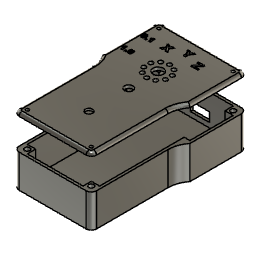
3018 pendant case (Autodesk Fusion 360 design; units mm, degrees)
Autodesk Fusion 360 part; units mm, degrees
note: some values were not read from the file. Chosen so that the rebuilt part matches the saved one: the layout of a text. Set by a fixed rule: which sketch regions a step uses.
sketch "Sketch1" plane through (0, 0, 0) normal (0, 0, 1) x (1, 0, 0)
  line L0 (35, -45) -> (-35, -45)
  line L1 (-35, -45) -> (-35, 45)
  line L2 (35, 45) -> (35, -45)
  line L3 (35, -45) -> (-35, 45) construction
  line L4 (-35, -45) -> (35, 45) construction
  line L5 (-35, 45) -> (-39.456, 45)
  line L6 (-39.456, 45) -> (-39.456, 95)
  line L7 (-39.456, 95) -> (40.544, 95)
  line L8 (40.544, 95) -> (40.544, 45)
  line L9 (40.544, 45) -> (35, 45)
  line L10 (43.044, 42.5) -> (37.5, 42.5)
  line L11 (37.5, 42.5) -> (37.5, -47.5)
  line L12 (37.5, -47.5) -> (-37.5, -47.5)
  line L13 (-37.5, -47.5) -> (-37.5, 42.5)
  line L14 (-37.5, 42.5) -> (-41.956, 42.5)
  line L15 (-41.956, 42.5) -> (-41.956, 97.5)
  line L16 (-41.956, 97.5) -> (43.044, 97.5)
  line L17 (43.044, 97.5) -> (43.044, 42.5)
  dimension "d2" = 90
  dimension "d4" = 50
  dimension "d5" = 80
  dimension "d6" = 50
  dimension "d7" = -2.5
  dimension "d160" = 70
  constraint horizontal L0
  constraint perpendicular L0 L1
  constraint parallel L1 L2
  constraint coincident L3 origin
  constraint coincident L4 origin
  constraint perpendicular L1 L5
  constraint perpendicular L6 L7
  constraint perpendicular L7 L8
  constraint perpendicular L2 L9
  constraint perpendicular L8 L9
  measures "d2" distance of L0.end L1.end
  measures "d4" distance of L5.end L6.end
  measures "d5" distance of L6.end L7.end
  measures "d6" distance of L7.end L8.end
  measures "d160" distance of L0.start L0.end
extrude "Extrude1" add sketch "Sketch1" along normal blind 2 contours L0 L1 L2 L5 L6 L7 L8 L9 makes body 1
extrude "Extrude2" add sketch "Sketch1" along normal blind 32 bodies 1
sketch "Sketch2" plane through (0, 0, 2) normal (0, 0, 1) x (-1, 0, 0)
  line L0 (-40.544, -45) -> (-40.544, -95)
  line L1 (-40.544, -95) -> (39.456, -95)
  line L2 (39.456, -95) -> (39.456, -45)
  line L3 (39.456, -45) -> (35, -45)
  line L4 (35, -45) -> (35, 45)
  line L5 (35, 45) -> (-35, 45)
  line L6 (-35, 45) -> (-35, -45)
  line L7 (-35, -45) -> (-40.544, -45)
  circle A0 centre (0, 10) radius 32.5
  line L8 (39.456, -95) -> (31.456, -95)
  line L9 (31.456, -95) -> (31.456, -87)
  line L10 (31.456, -87) -> (39.456, -87)
  line L11 (39.456, -87) -> (39.456, -95)
  line L12 (-40.544, -95) -> (-32.544, -95)
  line L13 (-32.544, -95) -> (-32.544, -87)
  line L14 (-32.544, -87) -> (-40.544, -87)
  line L15 (-40.544, -87) -> (-40.544, -95)
  line L16 (35, 45) -> (27, 45)
  line L17 (27, 45) -> (27, 37)
  line L18 (27, 37) -> (35, 37)
  line L19 (35, 37) -> (35, 45)
  line L20 (-35, 45) -> (-27, 45)
  line L21 (-27, 45) -> (-27, 37)
  line L22 (-27, 37) -> (-35, 37)
  line L23 (-35, 37) -> (-35, 45)
  dimension "d13" = 65
  dimension "d24" = 8
  dimension "d25" = 8
  dimension "d26" = 8
  dimension "d27" = 8
  dimension "d28" = 8
  dimension "d29" = 8
  dimension "d30" = 8
  dimension "d31" = 8
  constraint horizontal L8
  constraint vertical L9
  constraint horizontal L10
  constraint vertical L11
  constraint coincident L1.end L2.start
  constraint horizontal L12
  constraint vertical L13
  constraint horizontal L14
  constraint vertical L15
  constraint coincident L0.end L1.start
  constraint horizontal L16
  constraint vertical L17
  constraint horizontal L18
  constraint vertical L19
  constraint coincident L4.end L5.start
  constraint horizontal L20
  constraint vertical L21
  constraint horizontal L22
  constraint vertical L23
  constraint coincident L5.end L6.start
  measures "d13" diameter of A0
  measures "d24" distance of L1.end L8.end
  measures "d25" distance of L1.end L10.end
  measures "d26" distance of L0.end L12.end
  measures "d27" distance of L0.end L14.end
  measures "d28" distance of L4.end L16.end
  measures "d29" distance of L4.end L18.end
  measures "d30" distance of L5.end L20.end
  measures "d31" distance of L5.end L22.end
extrude "Extrude3" add sketch "Sketch2" along normal up to surface (30 mm away) contours L0 L1 L12 L13 L14 L15 | L5 L6 L20 L21 L22 L23 | L1 L2 L8 L9 L10 L11 | L4 L5 L16 L17 L18 L19 bodies 1
fillet "Fillet1" radius 5 4 edges at (37.5, -47.5, 16) (-37.5, -47.5, 16) (43.044, 97.5, 16) (-41.956, 97.5, 16) on bodies 1
fillet "Fillet7" radius 25 2 edges at (-37.5, 42.5, 16) (37.5, 42.5, 16) on bodies 1
fillet "Fillet2" [suppressed]
fillet "Fillet3" [suppressed]
sketch "Sketch3" plane through (0, 0, 32) normal (0, 0, 1) x (-1, 0, 0)
  arc A0 (36.956, -97.5) -> (41.956, -92.5) centre (36.956, -92.5) ccw
  line L0 (41.956, -92.5) -> (41.956, -42.5)
  line L1 (37.5, -42.5) -> (37.5, 42.5)
  arc A1 (37.5, 42.5) -> (32.5, 47.5) centre (32.5, 42.5) ccw
  line L2 (32.5, 47.5) -> (-32.5, 47.5)
  arc A2 (-32.5, 47.5) -> (-37.5, 42.5) centre (-32.5, 42.5) ccw
  line L3 (-37.5, 42.5) -> (-37.5, -42.5)
  line L4 (-43.044, -42.5) -> (-43.044, -92.5)
  arc A3 (-43.044, -92.5) -> (-38.044, -97.5) centre (-38.044, -92.5) ccw
  line L5 (-38.044, -97.5) -> (36.956, -97.5)
  line L6 (-40.544, -87) -> (-40.544, -45)
  line L7 (-40.544, -45) -> (-35, -45)
  line L8 (-35, -45) -> (-35, 37)
  line L9 (-35, 37) -> (-27, 37)
  line L10 (-27, 37) -> (-27, 45)
  line L11 (-27, 45) -> (27, 45)
  line L12 (27, 45) -> (27, 37)
  line L13 (27, 37) -> (35, 37)
  line L14 (35, 37) -> (35, -45)
  line L15 (35, -45) -> (39.456, -45)
  line L16 (39.456, -45) -> (39.456, -87)
  line L17 (39.456, -87) -> (31.456, -87)
  line L18 (31.456, -87) -> (31.456, -95)
  line L19 (31.456, -95) -> (-32.544, -95)
  line L20 (-32.544, -95) -> (-32.544, -87)
  line L21 (-32.544, -87) -> (-40.544, -87)
  circle A4 centre (35.456, -91) radius 2.5
  circle A5 centre (-36.544, -91) radius 2.5
  circle A6 centre (31, 41) radius 2.5
  circle A7 centre (-31, 41) radius 2.5
  line L22 (41.956, -42.5) -> (37.5, -42.5)
  line L23 (-37.5, -42.5) -> (-43.044, -42.5)
  dimension "d34" = 5
  dimension "d35" = 4
  dimension "d36" = 4
  dimension "d37" = 5
  dimension "d38" = 4
  dimension "d39" = 4
  dimension "d40" = 5
  dimension "d41" = 4
  dimension "d42" = 4
  dimension "d43" = 5
  dimension "d44" = 4
  dimension "d45" = 4
  measures "d34" diameter of A4
  measures "d35" distance of L17 A4.centre
  measures "d36" distance of L18 A4.centre
  measures "d37" diameter of A5
  measures "d38" distance of L20 A5.centre
  measures "d39" distance of L21 A5.centre
  measures "d40" diameter of A6
  measures "d41" distance of L13 A6.centre
  measures "d42" distance of L12 A6.centre
  measures "d43" diameter of A7
  measures "d44" distance of L10 A7.centre
  measures "d45" distance of L9 A7.centre
extrude "Extrude4" cut sketch "Sketch3" against normal blind 5.2 contours A4 | A5 | A6 | A7 bodies 1
ref_plane "WorkPlane1" through (0.544, 25, 62) normal (0, 0, 1) x (1, 0, 0)
sketch "Sketch4" plane through (0, 25, 62) normal (0, 0, 1) x (1, 0, 0)
  arc A0 (-36.956, 72.5) -> (-41.956, 67.5) centre (-36.956, 67.5) ccw
  line L0 (-36.956, 72.5) -> (38.044, 72.5)
  arc A1 (43.044, 67.5) -> (38.044, 72.5) centre (38.044, 67.5) ccw
  line L1 (43.044, 67.5) -> (43.044, 17.5)
  line L2 (37.5, 1.8009) -> (37.5, -67.5)
  arc A2 (32.5, -72.5) -> (37.5, -67.5) centre (32.5, -67.5) ccw
  line L3 (32.5, -72.5) -> (-32.5, -72.5)
  arc A3 (-37.5, -67.5) -> (-32.5, -72.5) centre (-32.5, -67.5) ccw
  line L4 (-37.5, -67.5) -> (-37.5, 3.2541)
  line L5 (-41.956, 17.5) -> (-41.956, 67.5)
  arc A4 (43.044, 17.5) -> (37.5, 1.8009) centre (62.5, 1.8009) ccw
  arc A5 (-37.5, 3.2541) -> (-41.956, 17.5) centre (-62.5, 3.2541) ccw
extrude "Extrude5" add sketch "Sketch4" along normal blind 3 separate body makes body 2
sketch "Sketch5" plane through (0, 0, 32) normal (0, 0, 1) x (1, 0, 0)
  circle A0 centre (36.544, 91) radius 2.5
  circle A1 centre (-35.456, 91) radius 2.5
  circle A2 centre (31, -41) radius 2.5
  circle A3 centre (-31, -41) radius 2.5
  circle A4 centre (-35.456, 91) radius 1.5
  circle A5 centre (36.544, 91) radius 1.5
  circle A6 centre (31, -41) radius 1.5
  circle A7 centre (-31, -41) radius 1.5
  circle A8 centre (36.544, 91) radius 2.5
  circle A9 centre (-31, -41) radius 2.5
  circle A10 centre (-35.456, 91) radius 2.5
  circle A11 centre (31, -41) radius 2.5
  arc A12 (-36.956, 97.5) -> (-41.956, 92.5) centre (-36.956, 92.5) ccw
  line L0 (-41.956, 92.5) -> (-41.956, 42.5)
  arc A13 (-37.5, 28.2541) -> (-41.956, 42.5) centre (-62.5, 28.2541) ccw
  line L1 (-37.5, 28.2541) -> (-37.5, -42.5)
  arc A14 (-37.5, -42.5) -> (-32.5, -47.5) centre (-32.5, -42.5) ccw
  line L2 (-32.5, -47.5) -> (32.5, -47.5)
  arc A15 (32.5, -47.5) -> (37.5, -42.5) centre (32.5, -42.5) ccw
  line L3 (37.5, -42.5) -> (37.5, 26.8009)
  arc A16 (43.044, 42.5) -> (37.5, 26.8009) centre (62.5, 26.8009) ccw
  line L4 (43.044, 42.5) -> (43.044, 92.5)
  arc A17 (43.044, 92.5) -> (38.044, 97.5) centre (38.044, 92.5) ccw
  line L5 (38.044, 97.5) -> (-36.956, 97.5)
  line L6 (40.544, 87) -> (40.544, 45)
  line L7 (40.544, 45) -> (35, 45)
  line L8 (35, 45) -> (35, -37)
  line L9 (35, -37) -> (27, -37)
  line L10 (27, -37) -> (27, -45)
  line L11 (27, -45) -> (-27, -45)
  line L12 (-27, -45) -> (-27, -37)
  line L13 (-27, -37) -> (-35, -37)
  line L14 (-35, -37) -> (-35, 45)
  line L15 (-35, 45) -> (-39.456, 45)
  line L16 (-39.456, 45) -> (-39.456, 87)
  line L17 (-39.456, 87) -> (-31.456, 87)
  line L18 (-31.456, 87) -> (-31.456, 95)
  line L19 (-31.456, 95) -> (32.544, 95)
  line L20 (32.544, 95) -> (32.544, 87)
  line L21 (32.544, 87) -> (40.544, 87)
  dimension "d141" = 3
  dimension "d142" = 3
  dimension "d143" = 3
  dimension "d144" = 3
  constraint concentric A1 A4
  constraint concentric A0 A5
  constraint concentric A2 A6
  constraint concentric A3 A7
  measures "d141" diameter of A4
  measures "d142" diameter of A5
  measures "d143" diameter of A6
  measures "d144" diameter of A7
extrude "Extrude7" cut sketch "Sketch5" along normal up to surface (33 mm away) contours A4 | A5 | A6 | A7 bodies 2
sketch "Sketch6" plane through (0, 0, 65) normal (0, 0, 1) x (-1, 0, 0)
  circle A0 centre (0, 12.2844) radius 30.6
  circle A1 centre (0, 12.2844) radius 33.6
  circle A2 centre (0, 12.2844) radius 3.5
  circle A3 centre (-31, 41) radius 1.5
  circle A4 centre (-36.544, -91) radius 1.5
  circle A5 centre (31, 41) radius 1.5
  circle A6 centre (35.456, -91) radius 1.5
  arc A7 (37.5, 42.5) -> (32.5, 47.5) centre (32.5, 42.5) ccw
  line L0 (32.5, 47.5) -> (-32.5, 47.5)
  arc A8 (-32.5, 47.5) -> (-37.5, 42.5) centre (-32.5, 42.5) ccw
  line L1 (-37.5, 42.5) -> (-37.5, -26.8009)
  arc A9 (-43.044, -42.5) -> (-37.5, -26.8009) centre (-62.5, -26.8009) ccw
  line L2 (-43.044, -42.5) -> (-43.044, -92.5)
  arc A10 (-43.044, -92.5) -> (-38.044, -97.5) centre (-38.044, -92.5) ccw
  line L3 (-38.044, -97.5) -> (36.956, -97.5)
  arc A11 (36.956, -97.5) -> (41.956, -92.5) centre (36.956, -92.5) ccw
  line L4 (41.956, -92.5) -> (41.956, -42.5)
  arc A12 (37.5, -28.2541) -> (41.956, -42.5) centre (62.5, -28.2541) ccw
  line L5 (37.5, -28.2541) -> (37.5, 42.5)
  dimension "d57" = 61.2
  dimension "d58" = 3
  dimension "d62" = 7
  constraint concentric A0 A2
  measures "d57" diameter of A0
  measures "d62" diameter of A2
fillet "Fillet6" radius 3 12 edges at (-38.64, 35.7174, 65) (-37.5, -7.123, 65) (-36.0355, -46.0355, 65) (0, -47.5, 65) (36.0355, -46.0355, 65) (37.5, -7.8496, 65) (38.9267, 35.1255, 65) (43.044, 67.5, 65) (41.5795, 96.0355, 65) (0.544, 97.5, 65) (-40.4916, 96.0355, 65) (-41.956, 67.5, 65) on bodies 2
sketch "Sketch10" plane through (0, 0, 0) normal (0, 0, -1) x (1, 0, 0)
  line L0 (-47.5, -83.9701, -14.6252) -> (-47.5, -71.3701, -14.6252)
  line L1 (-47.5, -71.3701, -14.6252) -> (-47.5, -71.3701, -27.2252)
  line L2 (-47.5, -71.3701, -27.2252) -> (-47.5, -83.9701, -27.2252)
  line L3 (-47.5, -83.9701, -27.2252) -> (-47.5, -83.9701, -14.6252)
  line L4 (-47.5, -71.3701, -26.2252) -> (-47.5, -71.6701, -26.2252)
  line L5 (-47.5, -71.6701, -26.2252) -> (-47.5, -71.6701, -24.0252)
  line L6 (-47.5, -71.6701, -24.0252) -> (-47.5, -71.3701, -24.0252)
  line L7 (-47.5, -71.3701, -24.0252) -> (-47.5, -71.3701, -26.2252)
  line L8 (-47.5, -71.3701, -17.8252) -> (-47.5, -71.6701, -17.8252)
  line L9 (-47.5, -71.6701, -17.8252) -> (-47.5, -71.6701, -15.6252)
  line L10 (-47.5, -71.6701, -15.6252) -> (-47.5, -71.3701, -15.6252)
  line L11 (-47.5, -71.3701, -15.6252) -> (-47.5, -71.3701, -17.8252)
  line L12 (-47.5, -83.9701, -15.6252) -> (-47.5, -83.6701, -15.6252)
  line L13 (-47.5, -83.6701, -15.6252) -> (-47.5, -83.6701, -17.8252)
  line L14 (-47.5, -83.6701, -17.8252) -> (-47.5, -83.9701, -17.8252)
  line L15 (-47.5, -83.9701, -17.8252) -> (-47.5, -83.9701, -15.6252)
  line L16 (-47.5, -83.9701, -26.2252) -> (-47.5, -83.6701, -26.2252)
  line L17 (-47.5, -83.6701, -26.2252) -> (-47.5, -83.6701, -24.0252)
  line L18 (-47.5, -83.6701, -24.0252) -> (-47.5, -83.9701, -24.0252)
  line L19 (-47.5, -83.9701, -24.0252) -> (-47.5, -83.9701, -26.2252)
  line L20 (-47.5, -51.3701, -14.6252) -> (-47.5, -51.3701, -27.2252)
  line L21 (-47.5, -51.3701, -24.0252) -> (-47.5, -51.3701, -26.2252)
  line L22 (-47.5, -51.6701, -26.2252) -> (-47.5, -51.6701, -24.0252)
  line L23 (-47.5, -63.9701, -17.8252) -> (-47.5, -63.9701, -15.6252)
  line L24 (-47.5, -51.6701, -15.6252) -> (-47.5, -51.3701, -15.6252)
  line L25 (-47.5, -63.6701, -17.8252) -> (-47.5, -63.9701, -17.8252)
  line L26 (-47.5, -51.3701, -17.8252) -> (-47.5, -51.6701, -17.8252)
  line L27 (-47.5, -63.9701, -24.0252) -> (-47.5, -63.9701, -26.2252)
  line L28 (-47.5, -63.6701, -15.6252) -> (-47.5, -63.6701, -17.8252)
  line L29 (-47.5, -51.6701, -24.0252) -> (-47.5, -51.3701, -24.0252)
  line L30 (-47.5, -63.9701, -27.2252) -> (-47.5, -63.9701, -14.6252)
  line L31 (-47.5, -63.9701, -15.6252) -> (-47.5, -63.6701, -15.6252)
  line L32 (-47.5, -63.9701, -14.6252) -> (-47.5, -51.3701, -14.6252)
  line L33 (-47.5, -51.3701, -15.6252) -> (-47.5, -51.3701, -17.8252)
  line L34 (-47.5, -51.6701, -17.8252) -> (-47.5, -51.6701, -15.6252)
  line L35 (-47.5, -63.6701, -24.0252) -> (-47.5, -63.9701, -24.0252)
  line L36 (-47.5, -63.9701, -26.2252) -> (-47.5, -63.6701, -26.2252)
  line L37 (-47.5, -63.6701, -26.2252) -> (-47.5, -63.6701, -24.0252)
  line L38 (-47.5, -51.3701, -26.2252) -> (-47.5, -51.6701, -26.2252)
  line L39 (-47.5, -51.3701, -27.2252) -> (-47.5, -63.9701, -27.2252)
  arc A0 (-41.956, -92.5) -> (-36.956, -97.5) centre (-36.956, -92.5) ccw
  line L40 (-36.956, -97.5) -> (38.044, -97.5)
  arc A1 (38.044, -97.5) -> (43.044, -92.5) centre (38.044, -92.5) ccw
  line L41 (43.044, -92.5) -> (43.044, -42.5)
  line L42 (37.5, -26.8009) -> (37.5, 42.5)
  arc A2 (37.5, 42.5) -> (32.5, 47.5) centre (32.5, 42.5) ccw
  line L43 (32.5, 47.5) -> (-32.5, 47.5)
  arc A3 (-32.5, 47.5) -> (-37.5, 42.5) centre (-32.5, 42.5) ccw
  line L44 (-37.5, 42.5) -> (-37.5, -28.2541)
  line L45 (-41.956, -42.5) -> (-41.956, -92.5)
  arc A4 (37.5, -26.8009) -> (43.044, -42.5) centre (62.5, -26.8009) ccw
  arc A5 (-41.956, -42.5) -> (-37.5, -28.2541) centre (-62.5, -28.2541) ccw
  dimension "d104" = 12.6
  dimension "d105" = 12.6
  dimension "d106" = 0.3
  dimension "d107" = 2.2
  dimension "d108" = 1
  dimension "d109" = 0.3
  dimension "d110" = 2.2
  dimension "d111" = 1
  dimension "d112" = 0.3
  dimension "d113" = 2.2
  dimension "d114" = 1
  dimension "d115" = 0.3
  dimension "d116" = 2.2
  dimension "d117" = 1
  dimension "d118" = 12.6
  dimension "d119" = 12.6
  dimension "d120" = 0.3
  dimension "d121" = 2.2
  dimension "d122" = 1
  dimension "d123" = 0.3
  dimension "d124" = 2.2
  dimension "d125" = 1
  dimension "d126" = 0.3
  dimension "d127" = 2.2
  dimension "d128" = 1
  dimension "d129" = 0.3
  dimension "d130" = 2.2
  dimension "d131" = 1
sketch "Sketch10 (curves on the plane with normal 1, 0, 0 at -47.5 mm)" plane through (-47.5, 0, 0) normal (1, 0, 0) x (0, -1, 0)
  line L0 (-83.9701, -14.6252) -> (-71.3701, -14.6252)
  line L1 (-71.3701, -14.6252) -> (-71.3701, -27.2252)
  line L2 (-71.3701, -27.2252) -> (-83.9701, -27.2252)
  line L3 (-83.9701, -27.2252) -> (-83.9701, -14.6252)
  line L4 (-71.3701, -26.2252) -> (-71.6701, -26.2252)
  line L5 (-71.6701, -26.2252) -> (-71.6701, -24.0252)
  line L6 (-71.6701, -24.0252) -> (-71.3701, -24.0252)
  line L7 (-71.3701, -24.0252) -> (-71.3701, -26.2252)
  line L8 (-71.3701, -17.8252) -> (-71.6701, -17.8252)
  line L9 (-71.6701, -17.8252) -> (-71.6701, -15.6252)
  line L10 (-71.6701, -15.6252) -> (-71.3701, -15.6252)
  line L11 (-71.3701, -15.6252) -> (-71.3701, -17.8252)
  line L12 (-83.9701, -15.6252) -> (-83.6701, -15.6252)
  line L13 (-83.6701, -15.6252) -> (-83.6701, -17.8252)
  line L14 (-83.6701, -17.8252) -> (-83.9701, -17.8252)
  line L15 (-83.9701, -17.8252) -> (-83.9701, -15.6252)
  line L16 (-83.9701, -26.2252) -> (-83.6701, -26.2252)
  line L17 (-83.6701, -26.2252) -> (-83.6701, -24.0252)
  line L18 (-83.6701, -24.0252) -> (-83.9701, -24.0252)
  line L19 (-83.9701, -24.0252) -> (-83.9701, -26.2252)
  line L20 (-51.3701, -14.6252) -> (-51.3701, -27.2252)
  line L21 (-51.3701, -24.0252) -> (-51.3701, -26.2252)
  line L22 (-51.6701, -26.2252) -> (-51.6701, -24.0252)
  line L23 (-63.9701, -17.8252) -> (-63.9701, -15.6252)
  line L24 (-51.6701, -15.6252) -> (-51.3701, -15.6252)
  line L25 (-63.6701, -17.8252) -> (-63.9701, -17.8252)
  line L26 (-51.3701, -17.8252) -> (-51.6701, -17.8252)
  line L27 (-63.9701, -24.0252) -> (-63.9701, -26.2252)
  line L28 (-63.6701, -15.6252) -> (-63.6701, -17.8252)
  line L29 (-51.6701, -24.0252) -> (-51.3701, -24.0252)
  line L30 (-63.9701, -27.2252) -> (-63.9701, -14.6252)
  line L31 (-63.9701, -15.6252) -> (-63.6701, -15.6252)
  line L32 (-63.9701, -14.6252) -> (-51.3701, -14.6252)
  line L33 (-51.3701, -15.6252) -> (-51.3701, -17.8252)
  line L34 (-51.6701, -17.8252) -> (-51.6701, -15.6252)
  line L35 (-63.6701, -24.0252) -> (-63.9701, -24.0252)
  line L36 (-63.9701, -26.2252) -> (-63.6701, -26.2252)
  line L37 (-63.6701, -26.2252) -> (-63.6701, -24.0252)
  line L38 (-51.3701, -26.2252) -> (-51.6701, -26.2252)
  line L39 (-51.3701, -27.2252) -> (-63.9701, -27.2252)
extrude "Extrude15" cut sketch "Sketch10 (curves on the plane with normal 1, 0, 0 at -47.5 mm)" along normal up to surface (8.044 mm away) contours L0 L1 L2 L3 L4 L5 L6 L8 L9 L10 L12 L13 L14 L16 L17 L18 | L20 L22 L24 L25 L26 L28 L29 L30 L31 L32 L34 L35 L36 L37 L38 L39 bodies 1
sketch "XYZ Switch" plane through (0, 0, 65) normal (0, 0, 1) x (-1, 0, 0)
  circle A0 centre (0, -54.7981) radius 11
  circle A1 centre (0, -65.7981) radius 2.1
  circle A2 centre (6.4656, -63.6973) radius 2.1
  circle A3 centre (10.4616, -58.1973) radius 2.1
  circle A4 centre (10.4616, -51.3989) radius 2.1
  circle A5 centre (6.4656, -45.8989) radius 2.1
  circle A6 centre (0, -43.7981) radius 2.1
  circle A7 centre (-6.4656, -45.8989) radius 2.1
  circle A8 centre (-10.4616, -51.3989) radius 2.1
  circle A9 centre (-10.4616, -58.1973) radius 2.1
  circle A10 centre (-6.4656, -63.6973) radius 2.1
  circle A11 centre (0, -54.7981) radius 5.05
  circle A12 centre (-31, 41) radius 1.5
  circle A13 centre (-36.544, -91) radius 1.5
  circle A14 centre (31, 41) radius 1.5
  circle A15 centre (35.456, -91) radius 1.5
  arc A16 (34.5, -28.2541) -> (38.956, -43.4094) centre (62.5, -28.2541) ccw
  line L0 (34.5, -28.2541) -> (34.5, 42.5)
  arc A17 (34.5, 42.5) -> (32.5, 44.5) centre (32.5, 42.5) ccw
  line L1 (32.5, 44.5) -> (-32.5, 44.5)
  arc A18 (-32.5, 44.5) -> (-34.5, 42.5) centre (-32.5, 42.5) ccw
  line L2 (-34.5, 42.5) -> (-34.5, -26.8009)
  arc A19 (-40.044, -43.5259) -> (-34.5, -26.8009) centre (-62.5, -26.8009) ccw
  line L3 (-40.044, -43.5259) -> (-40.044, -92.5)
  arc A20 (-40.044, -92.5) -> (-38.044, -94.5) centre (-38.044, -92.5) ccw
  line L4 (-38.044, -94.5) -> (36.956, -94.5)
  arc A21 (36.956, -94.5) -> (38.956, -92.5) centre (36.956, -92.5) ccw
  line L5 (38.956, -92.5) -> (38.956, -43.4094)
  dimension "d134" = 22
  dimension "d135" = 4.2
  dimension "d137" = 360
  dimension "d140" = 10.1
  constraint coincident A0 A1.centre
  constraint concentric A0 A11
  measures "d134" diameter of A0
  measures "d135" diameter of A1
  measures "d140" diameter of A11
extrude "Extrude17" cut sketch "XYZ Switch" against normal up to surface (3 mm away) contours A0 A4 | A0 A4 | A0 A3 | A0 A3 | A0 A5 | A0 A5 | A0 A2 | A0 A2 | A0 A6 | A0 A6 | A0 A1 | A0 A1 | A0 A7 | A0 A7 | A0 A10 | A0 A10 | A0 A8 | A0 A8 | A0 A9 | A0 A9 | A11 bodies 2
extrude "Extrude18" cut sketch "Sketch6" against normal up to surface (3 mm away) contours A2 bodies 2
sketch "Sketch12" plane through (0, 25, 62) normal (0, 0, -1) x (1, 0, 0)
  line L0 (6.1, 31.4691) -> (-6.1, 31.4691)
  line L1 (-6.1, 31.4691) -> (-6.1, 43.6691)
  line L2 (-6.1, 43.6691) -> (6.1, 43.6691)
  line L3 (6.1, 43.6691) -> (6.1, 31.4691)
  line L4 (6.1, 31.4691) -> (-6.1, 43.6691) construction
  line L5 (-6.1, 31.4691) -> (6.1, 43.6691) construction
  circle A0 centre (0, 37.2844) radius 3.5
  circle A1 centre (-10.4616, -26.3989) radius 2.1
  circle A2 centre (6.4656, -38.6973) radius 2.1
  circle A3 centre (0, -18.7981) radius 2.1
  circle A4 centre (10.4616, -33.1973) radius 2.1
  circle A5 centre (-10.4616, -33.1973) radius 2.1
  circle A6 centre (-6.4656, -20.8989) radius 2.1
  circle A7 centre (0, -40.7981) radius 2.1
  circle A8 centre (6.4656, -20.8989) radius 2.1
  circle A9 centre (10.4616, -26.3989) radius 2.1
  circle A10 centre (-6.4656, -38.6973) radius 2.1
  circle A11 centre (0, -29.7981) radius 5.05
  circle A12 centre (31, 66) radius 1.5
  circle A13 centre (36.544, -66) radius 1.5
  circle A14 centre (-31, 66) radius 1.5
  circle A15 centre (-35.456, -66) radius 1.5
  arc A16 (-32.5, 72.5) -> (-37.5, 67.5) centre (-32.5, 67.5) ccw
  line L6 (-37.5, 67.5) -> (-37.5, -3.2541)
  arc A17 (-41.956, -17.5) -> (-37.5, -3.2541) centre (-62.5, -3.2541) ccw
  line L7 (-41.956, -17.5) -> (-41.956, -67.5)
  arc A18 (-41.956, -67.5) -> (-36.956, -72.5) centre (-36.956, -67.5) ccw
  line L8 (-36.956, -72.5) -> (38.044, -72.5)
  arc A19 (38.044, -72.5) -> (43.044, -67.5) centre (38.044, -67.5) ccw
  line L9 (43.044, -67.5) -> (43.044, -17.5)
  arc A20 (37.5, -1.8009) -> (43.044, -17.5) centre (62.5, -1.8009) ccw
  line L10 (37.5, -1.8009) -> (37.5, 67.5)
  arc A21 (37.5, 67.5) -> (32.5, 72.5) centre (32.5, 67.5) ccw
  line L11 (32.5, 72.5) -> (-32.5, 72.5)
  point P0 (0, 37.5691)
  dimension "d150" = 12.2
  dimension "d151" = 12.2
  constraint horizontal L0
  constraint perpendicular L0 L1
  constraint parallel L0 L2
  constraint parallel L1 L3
  constraint coincident L4 P0
  constraint coincident L5 P0
  measures "d150" distance of L1.end L2.end
  measures "d151" distance of L0.end L1.end
extrude "Extrude20" cut sketch "Sketch12" against normal blind 1 contours L0 L1 L2 L3 | A0 bodies 2
sketch "Sketch13" plane through (0, 97.5, 0) normal (0, 1, 0) x (-1, 0, 0)
  line L0 (36.956, 0) -> (36.956, 32)
  line L1 (36.956, 32) -> (-38.044, 32)
  line L2 (-38.044, 32) -> (-38.044, 0)
  line L3 (9, 6.5935) -> (-9.5, 6.5935)
  line L4 (-9.5, 6.5935) -> (-9.5, 15.5935)
  line L5 (-9.5, 15.5935) -> (9, 15.5935)
  line L6 (9, 15.5935) -> (9, 6.5935)
  line L7 (9, 6.5935) -> (-9.5, 15.5935) construction
  line L8 (-9.5, 6.5935) -> (9, 15.5935) construction
  line L9 (-38.044, 0) -> (36.956, 0)
  point P0 (-0.25, 11.0935)
  dimension "d156" = 18.5
  dimension "d157" = 9
  constraint horizontal L3
  constraint perpendicular L3 L4
  constraint parallel L3 L5
  constraint parallel L4 L6
  constraint coincident L7 P0
  constraint coincident L8 P0
  measures "d156" distance of L4.end L5.end
  measures "d157" distance of L3.end L4.end
extrude "Extrude21" cut sketch "Sketch13" against normal up to surface (2.5 mm away) contours L3 L4 L5 L6 bodies 1
sketch "Sketch14" plane through (0, 0, 65) normal (0, 0, 1) x (-1, 0, 0)
  circle A0 centre (0, 12.2844) radius 3.5
  circle A1 centre (10.4616, -51.3989) radius 2.1
  circle A2 centre (-6.4656, -63.6973) radius 2.1
  circle A3 centre (0, -43.7981) radius 2.1
  circle A4 centre (-10.4616, -58.1973) radius 2.1
  circle A5 centre (10.4616, -58.1973) radius 2.1
  circle A6 centre (6.4656, -45.8989) radius 2.1
  circle A7 centre (0, -65.7981) radius 2.1
  circle A8 centre (-6.4656, -45.8989) radius 2.1
  circle A9 centre (-10.4616, -51.3989) radius 2.1
  circle A10 centre (6.4656, -63.6973) radius 2.1
  circle A11 centre (0, -54.7981) radius 5.05
  circle A12 centre (35.456, -91) radius 1.5
  circle A13 centre (31, 41) radius 1.5
  circle A14 centre (-36.544, -91) radius 1.5
  circle A15 centre (-31, 41) radius 1.5
  circle A16 centre (0, 12.2844) radius 30
  arc A17 (34.5, -28.2541) -> (38.956, -43.4094) centre (62.5, -28.2541) ccw
  line L0 (34.5, -28.2541) -> (34.5, 42.5)
  arc A18 (34.5, 42.5) -> (32.5, 44.5) centre (32.5, 42.5) ccw
  line L1 (32.5, 44.5) -> (-32.5, 44.5)
  arc A19 (-32.5, 44.5) -> (-34.5, 42.5) centre (-32.5, 42.5) ccw
  line L2 (-34.5, 42.5) -> (-34.5, -26.8009)
  arc A20 (-40.044, -43.5259) -> (-34.5, -26.8009) centre (-62.5, -26.8009) ccw
  line L3 (-40.044, -43.5259) -> (-40.044, -92.5)
  arc A21 (-40.044, -92.5) -> (-38.044, -94.5) centre (-38.044, -92.5) ccw
  line L4 (-38.044, -94.5) -> (36.956, -94.5)
  arc A22 (36.956, -94.5) -> (38.956, -92.5) centre (36.956, -92.5) ccw
  line L5 (38.956, -92.5) -> (38.956, -43.4094)
  circle A23 centre (0, -54.7981) radius 20
  circle A24 centre (0, -26.2156) radius 4.05
  dimension "d161" = 60
  dimension "d166" = 40
  dimension "d167" = 8.1
  dimension "d168" = 38.5
  constraint concentric A0 A16
  constraint concentric A11 A23
  measures "d161" diameter of A16
  measures "d166" diameter of A23
  measures "d167" diameter of A24
  measures "d168" distance of A0.centre A24.centre
extrude "Extrude22" cut sketch "Sketch14" against normal up to surface (3 mm away) contours A24 bodies 2
sketch "tezxt" plane through (0, 0, 65) normal (0, 0, 1) x (-1, 0, 0)
  circle A0 centre (0, -26.2156) radius 4.05
  circle A1 centre (0, 12.2844) radius 3.5
  circle A2 centre (10.4616, -51.3989) radius 2.1
  circle A3 centre (-6.4656, -63.6973) radius 2.1
  circle A4 centre (0, -43.7981) radius 2.1
  circle A5 centre (-10.4616, -58.1973) radius 2.1
  circle A6 centre (10.4616, -58.1973) radius 2.1
  circle A7 centre (6.4656, -45.8989) radius 2.1
  circle A8 centre (0, -65.7981) radius 2.1
  circle A9 centre (-6.4656, -45.8989) radius 2.1
  circle A10 centre (-10.4616, -51.3989) radius 2.1
  circle A11 centre (6.4656, -63.6973) radius 2.1
  circle A12 centre (0, -54.7981) radius 5.05
  circle A13 centre (35.456, -91) radius 1.5
  circle A14 centre (31, 41) radius 1.5
  circle A15 centre (-36.544, -91) radius 1.5
  circle A16 centre (-31, 41) radius 1.5
  arc A17 (34.5, -28.2541) -> (38.956, -43.4094) centre (62.5, -28.2541) ccw
  line L0 (34.5, -28.2541) -> (34.5, 42.5)
  arc A18 (34.5, 42.5) -> (32.5, 44.5) centre (32.5, 42.5) ccw
  line L1 (32.5, 44.5) -> (-32.5, 44.5)
  arc A19 (-32.5, 44.5) -> (-34.5, 42.5) centre (-32.5, 42.5) ccw
  line L2 (-34.5, 42.5) -> (-34.5, -26.8009)
  arc A20 (-40.044, -43.5259) -> (-34.5, -26.8009) centre (-62.5, -26.8009) ccw
  line L3 (-40.044, -43.5259) -> (-40.044, -92.5)
  arc A21 (-40.044, -92.5) -> (-38.044, -94.5) centre (-38.044, -92.5) ccw
  line L4 (-38.044, -94.5) -> (36.956, -94.5)
  arc A22 (36.956, -94.5) -> (38.956, -92.5) centre (36.956, -92.5) ccw
  line L5 (38.956, -92.5) -> (38.956, -43.4094)
  line L6 (0, -54.7981) -> (0, -80)
  line L7 (0, -54.7981) -> (14.7893, -75.1539)
  circle A23 centre (0, -54.7981) radius 20
  line L8 (0, -54.7981) -> (-14.7893, -75.1539)
  line L9 (24.589, -75.6144) -> (-25, -75.6144) construction
  line L10 (18.7929, -75.6143) -> (11.034, -75.6144) construction
  line L11 (11.034, -75.6144) -> (11.0341, -82.1795) construction
  line L12 (11.0341, -82.1795) -> (18.793, -82.1795) construction
  line L13 (18.793, -82.1795) -> (18.7929, -75.6143) construction
  line L14 (-11.4575, -75.6041) -> (-20.128, -75.6144) construction
  line L15 (-20.128, -75.6144) -> (-20.1205, -81.9615) construction
  line L16 (-20.1205, -81.9615) -> (-11.4499, -81.9513) construction
  line L17 (-11.4499, -81.9513) -> (-11.4575, -75.6041) construction
  line L18 (3.7697, -84.9734) -> (-3.2303, -84.9734) construction
  line L19 (-3.2303, -84.9734) -> (-3.2303, -90.9734) construction
  line L20 (-3.2303, -90.9734) -> (3.7697, -90.9734) construction
  line L21 (3.7697, -90.9734) -> (3.7697, -84.9734) construction
  line L22 (38.456, -54.5561) -> (30.2541, -54.5561) construction
  line L23 (30.2541, -54.5561) -> (30.2541, -60.4782) construction
  line L24 (30.2541, -60.4782) -> (38.456, -60.4782) construction
  line L25 (38.456, -60.4782) -> (38.456, -54.5561) construction
  line L26 (38.5, -75.2) -> (28.5, -75.2) construction
  line L27 (28.5, -75.2) -> (28.5, -80.2) construction
  line L28 (28.5, -80.2) -> (38.5, -80.2) construction
  line L29 (38.5, -80.2) -> (38.5, -75.2) construction
  dimension "d171" = 36
  dimension "d172" = 40
  dimension "d173" = 36
  dimension "d174" = 7
  dimension "d176" = 7
  dimension "d177" = 7
  dimension "d180" = 5
  dimension "d181" = 5
  text T0 "X" font "Arial Black" height 7 align left top in box 7.7589 x 6.5652 at (18.7929, -75.6143) x (-1, -0.000009) y (0.000009, -1) spacing 1
  text T1 "Z" font "Arial Black" height 7 align left top in box 8.6706 x 6.3472 at (-11.4575, -75.6041) x (-0.999999, -0.001187) y (0.001187, -0.999999) spacing 1
  text T2 "Y" font "Arial Black" height 7 align left top in box 7 x 6 at (3.7697, -84.9734) x (-1, 0) y (0, -1) spacing 1 by line height
  text T3 "1.0" font "Arial Black" height 5 align left top in box 8.202 x 5.9221 at (38.456, -54.5561) x (-1, 0) y (0, -1) spacing 1
  text T4 "0.1\n" font "Arial Black" height 5 align left top in box 10 x 5 at (38.5, -75.2) x (-1, 0) y (0, -1) spacing 1
  constraint coincident A12.centre L6.start
  constraint vertical L6
  constraint horizontal L9
  constraint coincident L9
  measures "d171" angle of L6 L7
  measures "d172" diameter of A23
  measures "d173" angle of L6 L8
extrude "text" cut sketch "tezxt" against normal blind 1.5 text T0 T2 T1 T3 T4 bodies 2
equation "d168 = ( ( 67 / 2 ) * 1 mm ) + ( ( ( 30 - 20 ) / 2 ) * 1 mm )"
named bodies: "Bottom", "Top"
